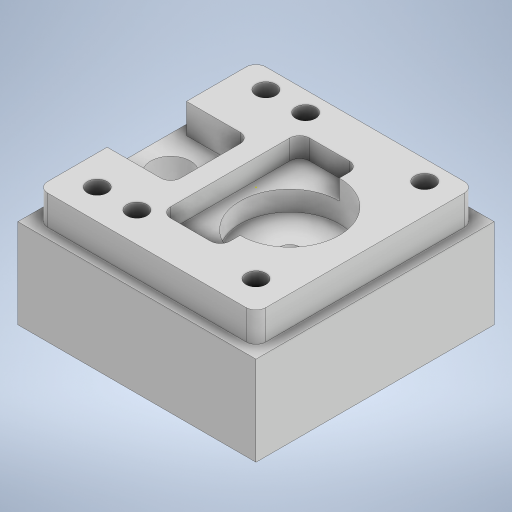
# Autodesk Inventor part: Exercise1
Saved by Autodesk Inventor 2023 (Build 270158000, 158)
## iProperties
Created: 2023-04-24
Part Number: Exercise1
Material: Generic
Document SubType Name: Modeling
Designer: dell
Density: 1 g/cm^3
Appearance: Default
Author: dell
Autodesk Inventor part; units mm, degrees
ref_plane "YZ Plane" through (0, 0, 0) normal (1, 0, 0) x (0, 1, 0)
ref_plane "XZ Plane" through (0, 0, 0) normal (0, 1, 0) x (-1, 0, 0)
ref_plane "XY Plane" through (0, 0, 0) normal (0, 0, 1) x (1, 0, 0)
sketch "Sketch1" plane through (0, 0, 0) normal (0, 1, 0) x (-1, 0, 0)
  line L0 (30, 30) -> (-30, 30)
  line L1 (-30, 30) -> (-30, -30)
  line L2 (-30, -30) -> (30, -30)
  line L3 (30, -30) -> (30, 30)
  line L4 (30, 30) -> (-30, -30) construction
  line L5 (-30, 30) -> (30, -30) construction
  point P0 (0, 0)
  dimension "d0" = 60
  dimension "d1" = 60
  constraints: 12 end point, 2 midpoint, 2 parallel, 1 horizontal, 1 perpendicular
  measures "d0" distance of L1.end L2.end
  measures "d1" distance of L2.end L0.start
extrude "Extrusion1" add sketch "Sketch1" along normal blind 22.5
sketch "Sketch2" plane through (0, 22.5, 0) normal (0, 1, 0) x (1, 0, 0)
  line L0 (-27.5, -27.5) -> (27.5, -27.5)
  line L1 (27.5, -27.5) -> (27.5, 27.5)
  line L2 (27.5, 27.5) -> (-27.5, 27.5)
  line L3 (-27.5, 27.5) -> (-27.5, -27.5)
  line L4 (-27.5, -27.5) -> (27.5, 27.5) construction
  line L5 (27.5, -27.5) -> (-27.5, 27.5) construction
  line L6 (30, 30) -> (-30, 30) projected
  line L7 (-30, 30) -> (-30, -30) projected
  point P0 (0, 0)
  dimension "d4" = 2.5
  dimension "d5" = 2.5
  constraints: 12 end point, 2 midpoint, 2 parallel, 1 horizontal, 1 perpendicular
  measures "d4" distance between parallel lines of L6 L2
  measures "d5" distance between parallel lines of L3 L7
extrude "Extrusion2" add sketch "Sketch2" along normal blind 7.5
sketch "Sketch5" plane through (0, 30, 0) normal (0, 1, 0) x (1, 0, 0)
  point P0 (0, 0)
sketch "Sketch6" plane through (0, 30, 0) normal (0, 1, 0) x (1, 0, 0)
  circle A0 centre (20, 22.5) radius 2.5
  circle A1 centre (-20, 22.5) radius 2.5
  line L0 (-30, -30) -> (30, -30) projected
  line L1 (30, -30) -> (30, 30) projected
  line L2 (-30, 30) -> (-30, -30) projected
  circle A2 centre (20, -20) radius 2.5
  circle A3 centre (-20, -20) radius 2.5
  line L3 (-27.5, -27.5) -> (27.5, -27.5) projected
  line L4 (27.5, 27.5) -> (-27.5, 27.5) projected
  circle A4 centre (-10, -20) radius 2.5
  circle A5 centre (-10, 22.5) radius 2.5
  point P0 (0, 0)
  dimension "d15" = 5
  dimension "d16" = 52.5
  dimension "d17" = 52.5
  dimension "d18" = 10
  dimension "d19" = 10
  dimension "d20" = 5
  dimension "d21" = 5
  dimension "d22" = 10
  dimension "d23" = 10
  dimension "d24" = 10
  dimension "d25" = 10
  dimension "d26" = 5
  dimension "d27" = 55
  dimension "d28" = 57.5
  dimension "d66" = 5
  dimension "d67" = 5
  dimension "d68" = 40
  dimension "d69" = 40
  constraints: 6 centre point
  measures "d15" diameter of A1
  measures "d16" distance from line of L0 A0.centre
  measures "d17" distance from line of L0 A1.centre
  measures "d18" distance from line of L1 A0.centre
  measures "d19" distance from line of L2 A1.centre
  measures "d20" diameter of A0
  measures "d21" diameter of A2
  measures "d22" distance from line of L0 A3.centre
  measures "d23" distance from line of L0 A2.centre
  measures "d24" distance from line of L2 A3.centre
  measures "d25" distance from line of L1 A2.centre
  measures "d26" diameter of A3
  measures "d27" distance between parallel lines of L3 L4
  measures "d28" distance between parallel lines of L0 L4
  measures "d66" diameter of A5
  measures "d67" diameter of A4
  measures "d68" distance from line of L1 A4.centre
  measures "d69" distance from line of L1 A5.centre
extrude "Extrusion5" cut sketch "Sketch6" against normal blind 10
sketch "Sketch7" plane through (0, 30, 0) normal (0, 1, 0) x (1, 0, 0)
  arc A0 (8.5, -12.5) -> (8.5, 12.5) centre (8.5, 0) ccw
  line L0 (30, -30) -> (30, 30) projected
  line L1 (8.5, 0) -> (8.5, 12.5)
  line L2 (8.5, 0) -> (8.5, -12.5)
  point P0 (0, 0)
  dimension "d32" = 21.5
  constraints: 4 end point, 2 point on circle, 2 vertical, 1 centre point
  measures "d32" distance from line of L0 L1.start
extrude "Extrusion6" cut sketch "Sketch7" against normal blind 10
sketch "Sketch8" plane through (0, 30, 0) normal (0, 1, 0) x (1, 0, 0)
  line L0 (-4, -17.5) -> (6, -17.5)
  line L1 (8.5, -15) -> (8.5, 15)
  line L2 (6, 17.5) -> (-4, 17.5)
  line L3 (-6.5, 15) -> (-6.5, -15)
  line L4 (-6.5, -17.5) -> (8.5, 17.5) construction
  line L5 (8.5, -17.5) -> (-6.5, 17.5) construction
  line L6 (30, -30) -> (30, 30) projected
  line L7 (8.5, -12.5) -> (8.5, 12.5) projected
  arc A0 (8.5, 12.5) -> (8.5, -12.5) centre (8.5, 0) ccw
  arc A1 (-4, 17.5) -> (-6.5, 15) centre (-4, 15) ccw
  arc A2 (8.5, 15) -> (6, 17.5) centre (6, 15) ccw
  arc A3 (-6.5, -15) -> (-4, -17.5) centre (-4, -15) ccw
  arc A4 (6, -17.5) -> (8.5, -15) centre (6, -15) ccw
  point P0 (0, 0)
  point P1 (1, 0)
  dimension "d35" = 35
  dimension "d37" = 21.5
  constraints: 14 end point, 10 point on circle, 8 tangent, 5 centre point, 3 midpoint, 2 parallel, 1 horizontal, 1 perpendicular
  measures "d35" distance of L5.end L4.start
  measures "d37" distance between parallel lines of L6 L1
extrude "Extrusion7" cut sketch "Sketch8" against normal blind 5
sketch "Sketch9" plane through (0, 25, 0) normal (0, 1, 0) x (1, 0, 0)
  line L0 (8.5, -12.5) -> (8.5, 12.5) projected
  arc A0 (8.5, 12.5) -> (8.5, -12.5) centre (8.5, 0) ccw
  line L1 (8.5, -12.5) -> (8.5, -15) projected
  line L2 (8.5, 15) -> (8.5, 12.5) projected
  line L3 (8.5, -12.5) -> (8.5, 12.5)
  point P0 (0, 0)
  constraints: 4 end point, 2 point on circle, 1 centre point, 1 midpoint, 1 vertical
extrude "Extrusion8" cut sketch "Sketch9" against normal blind 5
sketch "Sketch11" plane through (8.5, 20, 0) normal (0, 1, 0) x (1, 0, 0)
  circle A0 centre (0, 0) radius 2.5
  line L0 (21.5, -30) -> (21.5, 30) projected
  point P0 (-8.5, 0)
  dimension "d55" = 21.5
  dimension "d56" = 5
  constraints: 1 centre point
  measures "d55" distance from line of L0 A0.centre
  measures "d56" diameter of A0
extrude "Extrusion10" cut sketch "Sketch11" against normal blind 10
sketch "Sketch12" plane through (0, 30, 0) normal (0, 1, 0) x (1, 0, 0)
  line L0 (-27.5, -27.5) -> (-27.5, 27.5) projected
  line L1 (-27.5, 0) -> (-19.0189, 0)
  line L2 (-27.5, 10) -> (-27.5, -10)
  line L3 (-11.5, -7.5) -> (-11.5, 7.5)
  line L4 (-14, 10) -> (-27.5, 10)
  line L5 (-14, -10) -> (-27.5, -10)
  line L6 (30, -30) -> (30, 30) projected
  arc A0 (-11.5, 7.5) -> (-14, 10) centre (-14, 7.5) ccw
  arc A1 (-14, -10) -> (-11.5, -7.5) centre (-14, -7.5) ccw
  point P0 (0, 0)
  dimension "d59" = 20
  dimension "d60" = 10
  dimension "d61" = 41.5
  constraints: 10 end point, 4 point on circle, 4 tangent, 2 centre point, 2 horizontal, 2 point on line, 1 midpoint, 1 parallel, 1 vertical
  measures "d59" distance of L2.start L2.end
  measures "d60" distance from line of L2.end L1
  measures "d61" distance between parallel lines of L6 L3
extrude "Extrusion11" cut sketch "Sketch12" against normal blind 7.5
sketch "Sketch13" plane through (0, 30, 0) normal (0, 1, 0) x (1, 0, 0)
  point P0 (0, 0)
sketch "Sketch14" plane through (0, 22.5, 0) normal (0, 1, 0) x (1, 0, 0)
  circle A0 centre (-21.5, 0) radius 5
  line L0 (30, -30) -> (30, 30) projected
  point P0 (0, 0)
  dimension "d70" = 10
  dimension "d71" = 51.5
  constraints: 1 centre point
  measures "d70" diameter of A0
  measures "d71" distance from line of L0 A0.centre
extrude "Extrusion12" cut sketch "Sketch14" against normal blind 10
fillet "Fillet1" radius 2.5 1 edges at (-27.5, 26.25, -27.5)
fillet "Fillet2" radius 2.5 1 edges at (-27.5, 26.25, 27.5)
fillet "Fillet3" radius 2.5 1 edges at (27.5, 26.25, 27.5)
fillet "Fillet4" radius 2.5 1 edges at (27.5, 26.25, -27.5)
body "Solid1"
